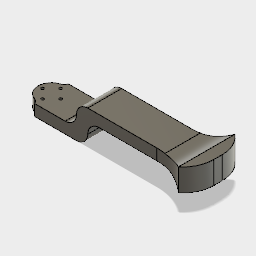
bracket4 v3 (Autodesk Fusion 360 design; units mm, degrees)
Autodesk Fusion 360 part; units mm, degrees
sketch "Sketch1" plane through (0, 0, 0) normal (0, 1, 0) x (1, 0, 0)
  line L0 (0, 0) -> (0, 8)
  circle A0 centre (0, 8) radius 1.2
  circle A1 centre (-8, 0) radius 1.2
  circle A2 centre (0, -8) radius 1.2
  circle A3 centre (8, 0) radius 1.2
  line L1 (0, 0) -> (0, 17)
  line L2 (0, 17) -> (-13, 17)
  line L3 (-13, 17) -> (37, 17)
  line L4 (37, 17) -> (37, -15)
  line L5 (37, -15) -> (-13, -15)
  line L6 (-13, -15) -> (-13, 17)
  line L7 (0, -8) -> (0, -15)
  circle A4 centre (0, 0) radius 12
  dimension "d1" = 8
  dimension "d2" = 2.4
  dimension "d4" = 360
  dimension "d5" = 17
  dimension "d6" = 32
  dimension "d7" = 50
  dimension "d8" = 24
  constraint coincident L0.start L1.start
  constraint perpendicular L1 L2
  constraint horizontal L3
  constraint vertical L4
  constraint horizontal L5
  constraint vertical L6
  constraint coincident L5 L0.start
  constraint perpendicular L5 L7
  measures "d2" diameter of A0
  measures "d8" diameter of A4
extrude "Extrude1" add sketch "Sketch1" along normal blind 10 contours L1 L3 L4 L5 L7 A4 | A4
sketch "Sketch2" plane through (0, 0, 0) normal (0, -1, 0) x (1, 0, 0)
  circle A0 centre (0, -8) radius 1.2
  circle A1 centre (0, 8) radius 1.2
  circle A2 centre (8, 0) radius 1.2
  circle A3 centre (-8, 0) radius 1.2
  arc A4 (0, 12) -> (0, -12) centre (0, 0) ccw
  line L0 (0, -12) -> (0, -17)
  line L1 (0, -17) -> (37, -17)
  line L2 (37, -17) -> (37, 15)
  line L3 (37, 15) -> (0, 15)
  line L4 (0, 15) -> (0, 12)
  line L5 (37, 15) -> (47, 15)
  line L6 (47, 15) -> (47, -17)
  line L7 (47, -17) -> (37, -17)
  line L8 (37, -17) -> (37, 15)
  dimension "d11" = 32
  constraint horizontal L5
  constraint vertical L6
  constraint horizontal L7
  constraint vertical L8
  constraint coincident A4.centre origin
extrude "Extrude2" add sketch "Sketch2" against normal blind 30 contours L2 L5 L6 L7 L8
sketch "Sketch3" plane through (47, 0, 0) normal (1, 0, 0) x (0, 0, -1)
  line L0 (-15, 0) -> (17, 0)
  line L1 (17, 0) -> (17, 30)
  line L2 (17, 30) -> (-15, 30)
  line L3 (-15, 30) -> (-15, 0)
  line L4 (-15, 30) -> (17, 30)
  line L5 (17, 30) -> (17, 20)
  line L6 (17, 20) -> (-15, 20)
  line L7 (-15, 20) -> (-15, 30)
  line L8 (17, 10) -> (17, 30)
  constraint horizontal L4
  constraint vertical L5
  constraint horizontal L6
  constraint vertical L7
  constraint midpoint origin L8
extrude "Extrude3" add sketch "Sketch3" along normal blind 100 contours L1 L2 L3 L4 L5 L6 L7 L8
sketch "Sketch4" plane through (0, 30, 0) normal (0, 1, 0) x (-1, 0, 0)
  line L0 (-147, -17) -> (-37, -17)
  line L1 (-37, -17) -> (-37, 15)
  line L2 (-37, 15) -> (-147, 15)
  line L3 (-147, 15) -> (-147, -17)
  line L4 (-147, -17) -> (-137, -17)
  line L5 (-137, -17) -> (-137, 15)
  line L6 (-137, 15) -> (-147, 15)
  line L7 (-147, 15) -> (-147, -17)
  dimension "d16" = 10
  dimension "d17" = 32
  constraint horizontal L4
  constraint vertical L5
  constraint horizontal L6
  constraint vertical L7
extrude "Extrude4" add sketch "Sketch4" along normal blind 5 contours L0 L2 L3 L4 L5 L6 L7
sketch "Sketch5" plane through (0, 20, 0) normal (0, -1, 0) x (1, 0, 0)
  line L0 (47, 15) -> (47, -17)
  line L1 (47, -17) -> (147, -17)
  line L2 (147, -17) -> (147, 15)
  line L3 (147, 15) -> (47, 15)
  line L4 (147, 15) -> (137, 15)
  line L5 (137, 15) -> (137, -17)
  line L6 (137, -17) -> (147, -17)
  line L7 (147, -17) -> (147, 15)
  dimension "d20" = 10
  dimension "d21" = 32
  constraint horizontal L4
  constraint vertical L5
  constraint horizontal L6
  constraint vertical L7
extrude "Extrude5" add sketch "Sketch5" along normal blind 5 contours L1 L2 L3 L4 L5 L6 L7
sketch "Sketch6" plane through (0, 0, -17) normal (0, 0, -1) x (-1, 0, 0)
  line L0 (-47, 0) -> (0, 0)
  line L1 (0, 0) -> (0, 10)
  line L2 (0, 10) -> (-37, 10)
  line L3 (-37, 10) -> (-37, 30)
  line L4 (-37, 30) -> (-137, 30)
  line L5 (-137, 30) -> (-137, 35)
  line L6 (-137, 35) -> (-147, 35)
  line L7 (-147, 35) -> (-147, 15)
  line L8 (-147, 15) -> (-137, 15)
  line L9 (-137, 15) -> (-137, 20)
  line L10 (-137, 20) -> (-47, 20)
  line L11 (-47, 20) -> (-47, 0)
  line L12 (-137, 30) -> (-137, 20)
  constraint coincident L0.end L1.start
extrude "Extrude8" cut 1 faces at (73.6667, 26.6667, -17) along direction (0, 0, 1) blind 2
sketch "Sketch7" plane through (0, 0, 15) normal (0, 0, 1) x (1, 0, 0)
  line L0 (0, 0) -> (47, 0)
  line L1 (47, 0) -> (47, 20)
  line L2 (47, 20) -> (137, 20)
  line L3 (137, 20) -> (137, 15)
  line L4 (137, 15) -> (147, 15)
  line L5 (147, 15) -> (147, 35)
  line L6 (147, 35) -> (137, 35)
  line L7 (137, 35) -> (137, 30)
  line L8 (137, 30) -> (37, 30)
  line L9 (37, 30) -> (37, 10)
  line L10 (37, 10) -> (0, 10)
  line L11 (0, 10) -> (0, 0)
  line L12 (137, 30) -> (137, 20)
  constraint coincident L0.start L11.end
extrude "Extrude7" add sketch "Sketch7" along normal blind 10 contours L3 L4 L5 L6 L7 L12
fillet "Fillet3" radius 10 1 edges at (37, 30, -1)
fillet "Fillet4" radius 10 1 edges at (47, 20, -1)
fillet "Fillet5" radius 10 1 edges at (37, 10, -1)
fillet "Fillet6" radius 10 1 edges at (47, 0, -1)
fillet "Fillet7" radius 5 2 edges at (0, 5, -12) (0, 5, 12)
sketch "Sketch8" plane through (0, 0, -15) normal (0, 0, -1) x (-1, 0, 0)
  arc A0 (-47, 10) -> (-37, 0) centre (-37, 10) ccw
  line L0 (-37, 0) -> (0, 0)
  line L1 (0, 0) -> (0, 10)
  line L2 (0, 10) -> (-27, 10)
  arc A1 (-37, 20) -> (-27, 10) centre (-27, 20) ccw
  arc A2 (-37, 20) -> (-47, 30) centre (-47, 20) ccw
  line L3 (-47, 30) -> (-137, 30)
  line L4 (-137, 30) -> (-137, 35)
  line L5 (-137, 35) -> (-147, 35)
  line L6 (-147, 35) -> (-147, 15)
  line L7 (-147, 15) -> (-137, 15)
  line L8 (-137, 15) -> (-137, 20)
  line L9 (-137, 20) -> (-57, 20)
  arc A3 (-47, 10) -> (-57, 20) centre (-57, 10) ccw
  line L10 (-137, 30) -> (-137, 20)
  constraint coincident L0.end L1.start
extrude "Extrude9" add sketch "Sketch8" along normal blind 10 contours L4 L5 L6 L7 L8 L10
fillet "Fillet8" radius 27.5 2 edges at (147, 25, -25) (147, 25, 25)
fillet "Fillet9" radius 47.5 4 edges at (137, 30, 0) (137, 20, 0) (137, 25, -15) (137, 25, 15)
